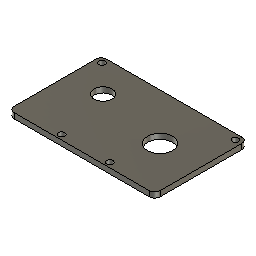
musti+babsi (Autodesk Fusion 360 design; units mm, degrees)
part number: 2026-07-21-17-44-04-627
Autodesk Fusion 360 part; units mm, degrees
sketch "Sketch1" plane through (0, 0, 0) normal (0, 0, 1) x (1, 0, 0)
  line L0 (3, 0) -> (79, 0)
  line L1 (82, 3) -> (82, 49)
  line L2 (79, 52) -> (3, 52)
  line L3 (0, 49) -> (0, 3)
  circle A0 centre (19, 34) radius 5
  circle A1 centre (59, 26) radius 7
  circle A2 centre (3.4233, 48.9343) radius 1.75
  line L4 (40.9233, 52) -> (40.9233, 0) construction
  arc A3 (3, 52) -> (0, 49) centre (3, 49) ccw
  arc A4 (82, 49) -> (79, 52) centre (79, 49) ccw
  arc A5 (79, 0) -> (82, 3) centre (79, 3) ccw
  arc A6 (0, 3) -> (3, 0) centre (3, 3) ccw
  circle A7 centre (78.4233, 48.9343) radius 1.75
  circle A8 centre (27, 2.7825) radius 1.75
  circle A9 centre (54, 2.7015) radius 1.75
  point P0 (82, 0)
  point P1 (0, 52)
  dimension "d1" = 82
  dimension "d2" = 52
  dimension "d3" = 10
  dimension "d4" = 18
  dimension "d5" = 19
  dimension "d6" = 14
  dimension "d7" = 26
  dimension "d8" = 23
  dimension "d9" = 3.5
  dimension "d10" = 3
  dimension "d11" = 3
  dimension "d12" = 3
  dimension "d13" = 3
  dimension "d14" = 75
  dimension "d15" = 3.5
  dimension "d16" = 27
  dimension "d17" = 3.5
  dimension "d18" = 54
  constraint horizontal L0
  constraint vertical L1
  constraint horizontal L2
  constraint vertical L3
  constraint perpendicular L2 L4
  constraint coincident L2 L4.start
  constraint coincident P1 L3
  constraint coincident P1 L2
  constraint tangent L3 A3
  constraint tangent L2 A3
  constraint tangent L2 A4
  constraint tangent L1 A4
  constraint coincident P0 L0
  constraint coincident P0 L1
  constraint tangent L0 A5
  constraint tangent L1 A5
  constraint coincident origin L0
  constraint coincident origin L3
  constraint tangent L0 A6
  constraint tangent L3 A6
  constraint symmetric A2 L4 A7
  measures "d1" distance of origin P0
  measures "d2" distance of origin P1
  measures "d3" diameter of A0
  measures "d4" distance of L2 A0.centre
  measures "d5" distance of L3 A0.centre
  measures "d6" diameter of A1
  measures "d7" distance of L2 A1.centre
  measures "d8" distance of L1 A1.centre
  measures "d9" diameter of A2
  measures "d10" radius of A3
  measures "d11" radius of A4
  measures "d12" radius of A5
  measures "d13" radius of A6
  measures "d14" distance of A2.centre A7.centre
  measures "d15" diameter of A8
  measures "d16" distance of L3 A8.centre
  measures "d17" diameter of A9
  measures "d18" distance of L3 A9.centre
extrude "Extrude1" add sketch "Sketch1" along normal blind 3
sketch "Sketch2" plane through (0, 0, 0) normal (0, 0, -1) x (1, 0, 0)
  circle A0 centre (59, -26) radius 7
  circle A1 centre (78.4233, -48.9343) radius 1.75
  circle A2 centre (3.4233, -48.9343) radius 1.75
  circle A3 centre (19, -34) radius 5
  circle A4 centre (27, -2.7825) radius 1.75
  circle A5 centre (54, -2.7015) radius 1.75
  arc A6 (3, 0) -> (0, -3) centre (3, -3) ccw
  line L0 (0, -3) -> (0, -49)
  arc A7 (0, -49) -> (3, -52) centre (3, -49) ccw
  line L1 (3, -52) -> (79, -52)
  arc A8 (79, -52) -> (82, -49) centre (79, -49) ccw
  line L2 (82, -49) -> (82, -3)
  arc A9 (82, -3) -> (79, 0) centre (79, -3) ccw
  line L3 (79, 0) -> (3, 0)
  line L4 (47, -7) -> (3, -7) construction
  line L5 (3, -7) -> (3, -27) construction
  line L6 (3, -27) -> (47, -27) construction
  line L7 (47, -27) -> (47, -7) construction
  spline S0 degree 5 poles (25, -17) (24.8982, -17.1954) (24.6862, -17.5626) (24.3433, -18.0433) (23.836, -18.5425) (23.1213, -18.9264) (22.3402, -19.0686) (21.5231, -18.9742) (20.7269, -18.6624) (20.0301, -18.1645) (19.5168, -17.5167) (19.2657, -16.7553) (19.3333, -15.9111) (19.7469, -15.006) (20.5162, -14.0555) (21.6391, -13.0691) (22.8144, -12.2556) (23.8484, -11.6327) (24.6049, -11.2118) (25, -11) knots 0 0 0 0 0 0 0.066667 0.133333 0.2 0.266667 0.333333 0.4 0.466667 0.533333 0.6 0.666667 0.733333 0.8 0.866667 0.933333 1 1 1 1 1 1
  line L8 (25, -7) -> (25, -19) construction
  spline S1 degree 5 poles (25, -17) (25.1018, -17.1954) (25.3138, -17.5626) (25.6567, -18.0433) (26.164, -18.5425) (26.8787, -18.9264) (27.6598, -19.0686) (28.4769, -18.9742) (29.2731, -18.6624) (29.9699, -18.1645) (30.4832, -17.5167) (30.7343, -16.7553) (30.6667, -15.9111) (30.2531, -15.006) (29.4838, -14.0555) (28.3609, -13.0691) (27.1856, -12.2556) (26.1516, -11.6327) (25.3951, -11.2118) (25, -11) knots 0 0 0 0 0 0 0.066667 0.133333 0.2 0.266667 0.333333 0.4 0.466667 0.533333 0.6 0.666667 0.733333 0.8 0.866667 0.933333 1 1 1 1 1 1
  line L9 (25.7459, -15.5691) -> (24.2541, -18.4309)
  line L10 (23.1131, -12.0117) -> (26.8869, -9.9883)
  line L11 (24.2541, -15.5691) -> (25.7459, -18.4309)
  line L12 (26.8869, -12.0117) -> (23.1131, -9.9883)
  spline S2 degree 3 poles (25, -18.7525) (24.6025, -19.1835) (24.136, -19.5246) (23.6175, -19.74) (22.5082, -20.2008) (21.2286, -20.0391) (20.1985, -19.4524) (19.3942, -18.9943) (18.693, -18.2593) (18.4347, -17.2901) (18.2166, -16.4717) (18.3743, -15.5495) (18.8324, -14.7253) (19.6448, -13.2633) (21.289, -11.9552) (23.6859, -10.5844) (23.9565, -10.4296) (24.237, -10.2744) (24.5275, -10.1187) (24.685, -10.0342) (24.8425, -9.9498) (25, -9.8653) knots 0.086991 0.086991 0.086991 0.086991 0.188377 0.188377 0.188377 0.405287 0.405287 0.405287 0.574651 0.574651 0.574651 0.71767 0.71767 0.71767 0.971359 0.971359 0.971359 1 1 1 1.015947 1.015947 1.015947 1.015947
  spline S3 degree 3 poles (25, -18.7525) (25.3975, -19.1835) (25.864, -19.5246) (26.3825, -19.74) (27.4918, -20.2008) (28.7714, -20.0391) (29.8015, -19.4524) (30.6058, -18.9943) (31.307, -18.2593) (31.5653, -17.2901) (31.7834, -16.4717) (31.6257, -15.5495) (31.1676, -14.7253) (30.3552, -13.2633) (28.711, -11.9552) (26.3141, -10.5844) (26.0435, -10.4296) (25.763, -10.2744) (25.4725, -10.1187) (25.315, -10.0342) (25.1575, -9.9498) (25, -9.8653) knots 0.086991 0.086991 0.086991 0.086991 0.188377 0.188377 0.188377 0.405287 0.405287 0.405287 0.574651 0.574651 0.574651 0.71767 0.71767 0.71767 0.971359 0.971359 0.971359 1 1 1 1.015947 1.015947 1.015947 1.015947
  point P0 (22, -19)
  point P1 (19.3926, -17)
  point P2 (28, -19)
  point P3 (30.6074, -17)
  dimension "d23" = 4
  dimension "d25" = 1
  text T0 "MUSTI + BABSI " font "Arial" height 4 bold align centre top in box 44 x 20 at (47, -7) x (-1, 0) y (0, -1) spacing 1
  constraint coincident L8.start
  constraint perpendicular L4 L8
  constraint midpoint S0.start L9
  constraint midpoint S0.end L10
  constraint symmetric S0.start L8 S1.start
  constraint symmetric P0 L8 P2
  constraint symmetric P1 L8 P3
  constraint symmetric S0.end L8 S1.end
  constraint symmetric L8 L9.start L11.start
  constraint symmetric L8 L9.end L11.end
  constraint symmetric L8 L10.start L12.start
  constraint symmetric L8 L10.end L12.end
extrude "Extrude2" cut sketch "Sketch2" sketch "Sketch2" against normal blind 1.5 contours L10 L12 S2 S3 | L10 L12 S2 S3 of sketch 2 text T0
equation "d24 = 'MUSTI + BABSI '"
